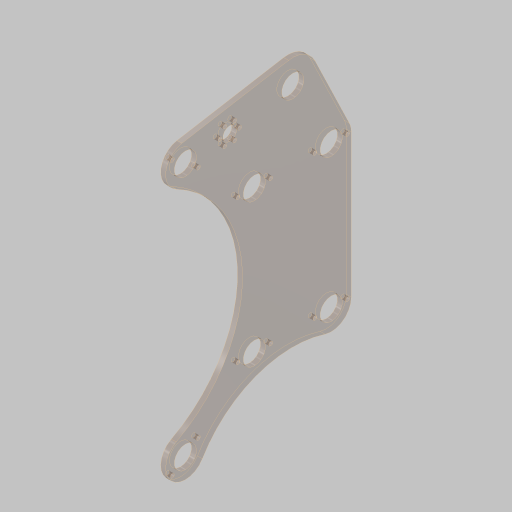
# Autodesk Inventor part: GP5-003
Saved by Autodesk Inventor 2023.5 (Build 275446000, 446)
## iProperties
Created: 2025-02-03
Part Number: GP5-003
Material: Polycarbonate, Smoke
Document SubType Name: Modeling
Designer: slick
Density: 1.2 g/cm^3
Appearance: Polycarbonate - Smoked
Author: slick
Autodesk Inventor part; units mm, degrees
ref_plane "YZ Plane" through (0, 0, 0) normal (1, 0, 0) x (0, 1, 0)
ref_plane "XZ Plane" through (0, 0, 0) normal (0, 1, 0) x (-1, 0, 0)
ref_plane "XY Plane" through (0, 0, 0) normal (0, 0, 1) x (1, 0, 0)
sketch "Sketch1" plane through (0, 0, 0) normal (1, 0, 0) x (0, 1, 0)
  line L0 (-12.7, 25.4) -> (12.7, 25.4) construction
  line L1 (12.7, 25.4) -> (12.7, -25.4) construction
  line L2 (12.7, -25.4) -> (-12.7, -25.4) construction
  line L3 (-12.7, -25.4) -> (-12.7, 25.4) construction
  line L4 (-12.7, 25.4) -> (12.7, -25.4) construction
  line L5 (12.7, 25.4) -> (-12.7, -25.4) construction
  circle A0 centre (-127, -49.4995) radius 38.1 construction
  circle A1 centre (-311.15, -49.4995) radius 38.1 construction
  circle A2 centre (-127, 49.4995) radius 38.1 construction
  circle A3 centre (-311.15, 49.4995) radius 38.1 construction
  line L6 (-127, -49.4995) -> (-127, 49.4995) construction
  line L7 (-311.15, -49.4995) -> (-311.15, 49.4995) construction
  line L8 (-161.925, -152.4) -> (-276.225, -152.4) construction
  line L9 (-276.225, -152.4) -> (-276.225, 152.4) construction
  line L10 (-276.225, 152.4) -> (-161.925, 152.4) construction
  line L11 (-161.925, 152.4) -> (-161.925, -152.4) construction
  line L12 (-161.925, -152.4) -> (-276.225, 152.4) construction
  line L13 (-276.225, -152.4) -> (-161.925, 152.4) construction
  circle A4 centre (-127, -49.4995) radius 34.925 construction
  circle A5 centre (-311.15, -49.4995) radius 34.925 construction
  circle A6 centre (-219.075, 279.4) radius 190.5 construction
  circle A7 centre (-55.6009, 138.3715) radius 25.4 construction
  circle A8 centre (-382.5491, 138.3715) radius 25.4 construction
  point P0 (0, 0)
  point P1 (-127, 0)
  point P2 (-311.15, 0)
  point P3 (-219.075, 0)
  dimension "d0" = 25.4
  dimension "d1" = 50.8
  dimension "d2" = 76.2
  dimension "d4" = 98.999
  dimension "d5" = 114.3
  dimension "d6" = 304.8
  dimension "d7" = 3.175
  dimension "d8" = 3.175
  dimension "d9" = 127
  dimension "d10" = 381
  dimension "d11" = 50.8
  dimension "d12" = 50.8
  dimension "d13" = 114.0003
  dimension "d14" = 279.4
  dimension "d35" = 49.4995
  constraints: 28 end point, 9 centre point, 6 horizontal alignment, 6 midpoint, 4 parallel, 4 tangent, 3 equal radius, 3 vertical alignment, 2 horizontal, 2 perpendicular, 2 vertical
  measures "d0" distance of L1.end L2.end
  measures "d1" distance of L0.end L1.end
  measures "d2" diameter of A0
  measures "d4" distance of L6.start L6.end
  measures "d5" distance of L9.end L10.end
  measures "d6" distance of L8.end L9.end
  measures "d7" radial gap between concentric circles of A0 A4
  measures "d8" radial gap between concentric circles of A1 A5
  measures "d9" distance from line of point (0, 0) L6
  measures "d10" diameter of A6
  measures "d11" diameter of A7
  measures "d12" diameter of A8
  measures "d13" distance of L6.end A7.centre
  measures "d14" distance of A6.centre point (-219.075, 0)
  measures "d35" distance of L6.start point (-127, 0)
sketch "Sketch2" plane through (0, 0, 0) normal (1, 0, 0) x (0, 1, 0)
  circle A0 centre (-127, -49.4995) radius 38.1 construction
  circle A1 centre (-127, 49.4995) radius 38.1 construction
  circle A2 centre (-127, -49.4995) radius 34.925 construction
  line L0 (-276.225, 152.4) -> (-161.925, 152.4) construction
  line L1 (-161.925, -152.4) -> (-276.225, -152.4) construction
  line L2 (-161.925, 152.4) -> (-161.925, -152.4) construction
  line L3 (-276.225, -152.4) -> (-161.925, 152.4) construction
  line L4 (-161.925, -152.4) -> (-276.225, 152.4) construction
  line L5 (-276.225, -152.4) -> (-276.225, 152.4) construction
  circle A3 centre (-311.15, 49.4995) radius 38.1 construction
  circle A4 centre (-311.15, -49.4995) radius 34.925 construction
  circle A5 centre (-311.15, -49.4995) radius 38.1 construction
  line L6 (-311.15, -49.4995) -> (-311.15, 49.4995) construction
  line L7 (-127, -49.4995) -> (-127, 49.4995) construction
  line L8 (-12.7, -25.4) -> (-12.7, 25.4) construction
  line L9 (12.7, 25.4) -> (12.7, -25.4) construction
  line L10 (12.7, -25.4) -> (-12.7, -25.4) construction
  line L11 (-12.7, 25.4) -> (12.7, -25.4) construction
  line L12 (12.7, 25.4) -> (-12.7, -25.4) construction
  line L13 (-12.7, 25.4) -> (12.7, 25.4) construction
  circle A6 centre (-219.075, 279.4) radius 190.5 construction
  circle A7 centre (-55.6009, 138.3715) radius 25.4 construction
  circle A8 centre (-382.5491, 138.3715) radius 25.4 construction
  circle A9 centre (-127, -49.4995) radius 14.2875
  circle A10 centre (-311.15, -49.4995) radius 14.2875
  circle A11 centre (-311.15, 49.4995) radius 14.2875
  circle A12 centre (-127, 49.4995) radius 14.2875
  circle A13 centre (-382.5491, 138.3715) radius 14.2875
  circle A14 centre (-55.6009, 138.3715) radius 14.2875
  circle A15 centre (-38.1, 0) radius 14.2875
  circle A16 centre (-38.1, 0) radius 39.3065 construction
  circle A17 centre (-38.1, 0) radius 25.4 construction
  circle A18 centre (-38.1, 0) radius 31.75 construction
  circle A19 centre (-127, -49.4995) radius 25.781 construction
  line L14 (-127, -70.518) -> (-127, -28.481) construction
  circle A20 centre (-127, -70.518) radius 4.7625 construction
  circle A21 centre (-311.15, -49.4995) radius 25.781 construction
  circle A22 centre (-311.15, 49.4995) radius 25.781 construction
  circle A23 centre (-127, 49.4995) radius 25.781 construction
  line L15 (-127, -75.2805) -> (-311.15, -75.2805)
  arc A24 (-335.6865, -41.5863) -> (-395.5081, 116.5261) centre (-464.6327, 0) ccw
  line L16 (-115.8012, -72.7212) -> (-24.3083, -28.5981)
  line L17 (-6.815, 5.4139) -> (-30.5729, 142.7026)
  arc A25 (-360.0409, 150.1419) -> (-78.1091, 150.1419) centre (-219.075, 223.8582) ccw
  arc A26 (-30.5729, 142.7026) -> (-78.1091, 150.1419) centre (-55.6009, 138.3715) ccw
  arc A27 (-360.0409, 150.1419) -> (-395.5081, 116.5261) centre (-382.5491, 138.3715) ccw
  arc A28 (-335.6865, -41.5863) -> (-311.15, -75.2805) centre (-311.15, -49.4995) ccw
  arc A29 (-127, -75.2805) -> (-115.8012, -72.7212) centre (-127, -49.4995) ccw
  arc A30 (-24.3083, -28.5981) -> (-6.815, 5.4139) centre (-38.1, 0) ccw
  circle A31 centre (-50.4775, 81.2215) radius 19.05 construction
  circle A32 centre (-50.4775, 81.2215) radius 12.7 construction
  circle A33 centre (-50.4775, 81.2215) radius 8.89
  line L18 (-311.15, 28.481) -> (-311.15, 70.518) construction
  line L19 (-311.15, -70.518) -> (-311.15, -28.481) construction
  line L20 (-68.3009, 121.6238) -> (-42.9009, 155.1193) construction
  line L21 (-369.8491, 121.6238) -> (-395.2491, 155.1193) construction
  line L22 (-127, 28.481) -> (-127, 70.518) construction
  point P0 (0, 0)
  point P1 (-127, 0)
  point P2 (-219.075, 0)
  point P3 (-311.15, 0)
  point P4 (0, 0)
  point P5 (-38.1, 25.4)
  point P6 (-50.4775, 68.5215)
  point P7 (-55.6009, 138.3715)
  point P8 (-39.479, 74.8715)
  point P9 (-39.479, 87.5715)
  point P10 (-50.4775, 93.9215)
  point P11 (-61.4761, 87.5715)
  point P12 (-61.4761, 74.8715)
  dimension "d18" = 50.8
  dimension "d32" = 9.525
  dimension "d37" = 25.4
  dimension "d15" = 28.575
  dimension "d16" = 38.1
  dimension "d17" = 78.613
  dimension "d19" = 6.35
  dimension "d31" = 42.037
  dimension "d36" = 38.1
  dimension "d38" = 17.78
  dimension "d43" = 82.837
  dimension "d44" = 57.15
  dimension "d50" = 12.7
  dimension "d51" = 12.7
  dimension "d61" = 360
  constraints: 25 point on circle, 22 centre point, 22 coincident, 18 end point, 11 tangent, 9 equal radius, 8 vertical alignment, 6 midpoint, 5 equal length, 2 horizontal, 1 collinear, 1 horizontal alignment, 1 point on line, 14 other
  measures "d15" diameter of A9
  measures "d16" distance of A15.centre point (0, 0)
  measures "d17" diameter of A16
  measures "d31" distance of L14.end L14.start
  measures "d36" diameter of A31
  measures "d38" diameter of A33
  measures "d43" distance of A1.centre A31.centre
  measures "d44" vertical distance of A7.centre point (-50.478, 81.222)
  measures "d50" horizontal distance of point (-55.601, 138.372) L20.start
  measures "d51" horizontal distance of A8.centre L21.start
extrude "Extrusion1" add sketch "Sketch2" along normal blind 6.35
hole "Hole1" at (0, -127, -49.4995) at (0, -127, 49.4995) at (0, -161.925, 152.4) at (0, -161.925, -152.4) at (0, -276.225, 152.4) at (0, -311.15, 49.4995) at (0, -311.15, -49.4995) at (0, -276.225, -152.4) at (0, -127, -70.518) at (0, -127, -28.481) at (0, -50.4775, 68.5215) at (0, -311.15, 28.481) at (0, -311.15, 70.518) at (0, -311.15, -70.518) at (0, -311.15, -28.481) at (0, -68.3009, 121.6238) at (0, -42.9009, 155.1193) at (0, -369.8491, 121.6238) at (0, -395.2491, 155.1193) at (0, -127, 28.481) at (0, -127, 70.518) at (0, -61.4761, 74.8715) at (0, -61.4761, 87.5715) at (0, -50.4775, 93.9215) at (0, -39.479, 87.5715) at (0, -39.479, 74.8715) direction (1, 0, 0) diameter 5.1054 end through all clearance for "Flat Head Machine Screw (82)" size "#10" standard "Ansi Unified Screw Threads"
equation "\"d51\" = d50"
body "Solid1"
